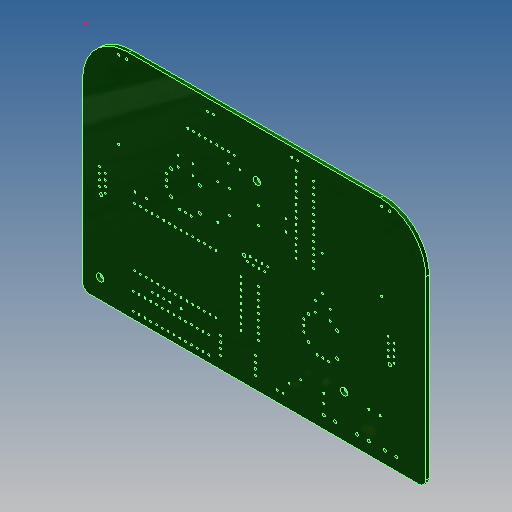
# Autodesk Inventor part: manette_2019.kicad_pcb_Contour
Saved by Autodesk Inventor 2019 (Build 230136000, 136)
## iProperties
Created: 2019-05-14
Part Number: manette_2019.kicad_pcb_Contour
Project: Nom Projet
Material: .
Description: Nom pièce
Document SubType Name: Modeling
Designer: Adel.KAHRIMANOVIC
Authority: brut Ø
Density: 0.001 g/cm^3
Appearance: Contour du circuit imprimé
Author: Adel.KAHRIMANOVIC
Material number: ---
Autodesk Inventor part; units mm, degrees
ref_plane "Plan YZ" through (0, 0, 0) normal (1, 0, 0) x (0, 1, 0)
ref_plane "Plan XZ" through (0, 0, 0) normal (0, 1, 0) x (-1, 0, 0)
ref_plane "Plan XY" through (0, 0, 0) normal (0, 0, 1) x (1, 0, 0)
sketch "Esquisse1" plane through (0, 0, 0) normal (0, 0, 1) x (1, 0, 0)
  point P0 (0, 0)
sketch "Esquisse6" plane through (0, 0, 0) normal (0, 0, 1) x (1, 0, 0)
  arc A0 (0, -97) -> (3, -100) centre (3, -97) ccw
  line L0 (3, -100) -> (147, -100)
  arc A1 (147, -100) -> (150, -97) centre (147, -97) ccw
  line L1 (150, -97) -> (150, -20)
  arc A2 (150, -20) -> (130, 0) centre (130, -20) ccw
  line L2 (130, 0) -> (20, 0)
  arc A3 (20, 0) -> (0, -20) centre (20, -20) ccw
  line L3 (0, -20) -> (0, -97)
  circle A4 centre (125.095, -82.55) radius 0.4
  circle A5 centre (130.095, -82.55) radius 0.4
  circle A6 centre (27.86, -51.435) radius 0.4
  circle A7 centre (22.86, -51.435) radius 0.4
  circle A8 centre (88.9, -28.575) radius 0.4
  circle A9 centre (88.9, -33.575) radius 0.4
  circle A10 centre (38.1165, -85.5345) radius 0.4
  circle A11 centre (43.1165, -85.5345) radius 0.4
  circle A12 centre (63.7667, -20.0406) radius 0.4
  circle A13 centre (68.7667, -20.0406) radius 0.4
  circle A14 centre (64.135, -29.5494) radius 0.4
  circle A15 centre (64.135, -39.7094) radius 0.4
  circle A16 centre (95.25, -86.36) radius 0.4
  circle A17 centre (105.41, -86.36) radius 0.4
  circle A18 centre (120.015, -94.615) radius 0.65
  circle A19 centre (125.095, -94.615) radius 0.65
  circle A20 centre (132.08, -94.615) radius 0.65
  circle A21 centre (137.16, -94.615) radius 0.65
  circle A22 centre (57.15, -5) radius 0.4
  circle A23 centre (54.61, -5) radius 0.4
  circle A24 centre (91.46, -4) radius 0.4
  circle A25 centre (94, -4) radius 0.4
  circle A26 centre (66.294, -15.748) radius 0.4
  circle A27 centre (63.754, -15.748) radius 0.4
  circle A28 centre (61.214, -15.748) radius 0.4
  circle A29 centre (58.674, -15.748) radius 0.4
  circle A30 centre (56.134, -15.748) radius 0.4
  circle A31 centre (53.594, -15.748) radius 0.4
  circle A32 centre (51.054, -15.748) radius 0.4
  circle A33 centre (48.514, -15.748) radius 0.4
  circle A34 centre (45.974, -15.748) radius 0.4
  circle A35 centre (105.41, -94.615) radius 0.65
  circle A36 centre (110.49, -94.615) radius 0.65
  circle A37 centre (87.63, -95.25) radius 0.4
  circle A38 centre (85.09, -95.25) radius 0.4
  circle A39 centre (136.144, -59.69) radius 0.4
  circle A40 centre (133.604, -58.42) radius 0.4
  circle A41 centre (136.144, -57.15) radius 0.4
  circle A42 centre (133.604, -55.88) radius 0.4
  circle A43 centre (136.144, -54.61) radius 0.4
  circle A44 centre (133.604, -53.34) radius 0.4
  circle A45 centre (136.144, -52.07) radius 0.4
  circle A46 centre (133.604, -50.8) radius 0.4
  circle A47 centre (9.906, -58.42) radius 0.4
  circle A48 centre (7.366, -57.15) radius 0.4
  circle A49 centre (9.906, -55.88) radius 0.4
  circle A50 centre (7.366, -54.61) radius 0.4
  circle A51 centre (9.906, -53.34) radius 0.4
  circle A52 centre (7.366, -52.07) radius 0.4
  circle A53 centre (9.906, -50.8) radius 0.4
  circle A54 centre (7.366, -49.53) radius 0.4
  circle A55 centre (80.9244, -50.73) radius 0.4
  circle A56 centre (79.6544, -53.27) radius 0.4
  circle A57 centre (78.3844, -50.73) radius 0.4
  circle A58 centre (77.1144, -53.27) radius 0.4
  circle A59 centre (75.8444, -50.73) radius 0.4
  circle A60 centre (74.5744, -53.27) radius 0.4
  circle A61 centre (73.3044, -50.73) radius 0.4
  circle A62 centre (72.0344, -53.27) radius 0.4
  circle A63 centre (36.75, -37.5) radius 0.45
  circle A64 centre (36.75, -40) radius 0.45
  circle A65 centre (36.75, -42.5) radius 0.45
  circle A66 centre (45, -48.25) radius 0.45
  circle A67 centre (42.5, -48.25) radius 0.45
  circle A68 centre (47.5, -48.25) radius 0.45
  circle A69 centre (41.75, -32.55) radius 0.4
  circle A70 centre (48.25, -32.55) radius 0.4
  circle A71 centre (48.25, -28.05) radius 0.4
  circle A72 centre (41.75, -28.05) radius 0.4
  circle A73 centre (101.75, -53.05) radius 0.4
  circle A74 centre (108.25, -53.05) radius 0.4
  circle A75 centre (108.25, -57.55) radius 0.4
  circle A76 centre (101.75, -57.55) radius 0.4
  circle A77 centre (107.5, -73.25) radius 0.45
  circle A78 centre (102.5, -73.25) radius 0.45
  circle A79 centre (105, -73.25) radius 0.45
  circle A80 centre (96.75, -67.5) radius 0.45
  circle A81 centre (96.75, -65) radius 0.45
  circle A82 centre (96.75, -62.5) radius 0.45
  circle A83 centre (76.835, -29.5494) radius 0.4
  circle A84 centre (76.835, -37.1694) radius 0.4
  circle A85 centre (90.17, -90.17) radius 0.4
  circle A86 centre (105.41, -90.17) radius 0.4
  circle A87 centre (59.055, -44.7894) radius 0.4
  circle A88 centre (59.055, -29.5494) radius 0.4
  circle A89 centre (104.775, -33.655) radius 0.4
  circle A90 centre (104.775, -48.895) radius 0.4
  circle A91 centre (15.75, -3) radius 0.5
  circle A92 centre (19.25, -3) radius 0.5
  circle A93 centre (15.75, -37) radius 0.5
  circle A94 centre (130.75, -3) radius 0.5
  circle A95 centre (134.25, -3) radius 0.5
  circle A96 centre (130.75, -37) radius 0.5
  circle A97 centre (37.975, -81.33) radius 0.4
  circle A98 centre (22.735, -81.33) radius 0.4
  circle A99 centre (53.215, -81.33) radius 0.4
  circle A100 centre (25.275, -81.33) radius 0.4
  circle A101 centre (40.515, -81.33) radius 0.4
  circle A102 centre (48.135, -81.33) radius 0.4
  circle A103 centre (27.815, -81.33) radius 0.4
  circle A104 centre (32.895, -81.33) radius 0.4
  circle A105 centre (43.055, -81.33) radius 0.4
  circle A106 centre (50.675, -81.33) radius 0.4
  circle A107 centre (55.755, -81.33) radius 0.4
  circle A108 centre (35.435, -81.33) radius 0.4
  circle A109 centre (45.595, -81.33) radius 0.4
  circle A110 centre (30.355, -81.33) radius 0.4
  circle A111 centre (58.295, -81.33) radius 0.4
  circle A112 centre (22.735, -55.83) radius 0.4
  circle A113 centre (25.275, -55.83) radius 0.4
  circle A114 centre (27.815, -55.83) radius 0.4
  circle A115 centre (30.355, -55.83) radius 0.4
  circle A116 centre (32.895, -55.83) radius 0.4
  circle A117 centre (35.435, -55.83) radius 0.4
  circle A118 centre (37.975, -55.83) radius 0.4
  circle A119 centre (40.515, -55.83) radius 0.4
  circle A120 centre (43.055, -55.83) radius 0.4
  circle A121 centre (45.595, -55.83) radius 0.4
  circle A122 centre (48.135, -55.83) radius 0.4
  circle A123 centre (50.675, -55.83) radius 0.4
  circle A124 centre (53.215, -55.83) radius 0.4
  circle A125 centre (55.755, -55.83) radius 0.4
  circle A126 centre (58.295, -55.83) radius 0.4
  circle A127 centre (55.1815, -96.9645) radius 0.4
  circle A128 centre (22.1615, -89.3445) radius 0.4
  circle A129 centre (52.6415, -96.9645) radius 0.4
  circle A130 centre (24.7015, -89.3445) radius 0.4
  circle A131 centre (50.1015, -96.9645) radius 0.4
  circle A132 centre (27.2415, -89.3445) radius 0.4
  circle A133 centre (47.5615, -96.9645) radius 0.4
  circle A134 centre (29.7815, -89.3445) radius 0.4
  circle A135 centre (45.0215, -96.9645) radius 0.4
  circle A136 centre (32.3215, -89.3445) radius 0.4
  circle A137 centre (42.4815, -96.9645) radius 0.4
  circle A138 centre (34.8615, -89.3445) radius 0.4
  circle A139 centre (39.9415, -96.9645) radius 0.4
  circle A140 centre (37.4015, -89.3445) radius 0.4
  circle A141 centre (37.4015, -96.9645) radius 0.4
  circle A142 centre (39.9415, -89.3445) radius 0.4
  circle A143 centre (34.8615, -96.9645) radius 0.4
  circle A144 centre (42.4815, -89.3445) radius 0.4
  circle A145 centre (32.3215, -96.9645) radius 0.4
  circle A146 centre (45.0215, -89.3445) radius 0.4
  circle A147 centre (29.7815, -96.9645) radius 0.4
  circle A148 centre (47.5615, -89.3445) radius 0.4
  circle A149 centre (27.2415, -96.9645) radius 0.4
  circle A150 centre (50.1015, -89.3445) radius 0.4
  circle A151 centre (24.7015, -96.9645) radius 0.4
  circle A152 centre (52.6415, -89.3445) radius 0.4
  circle A153 centre (22.1615, -96.9645) radius 0.4
  circle A154 centre (55.1815, -89.3445) radius 0.4
  circle A155 centre (93.345, -8.255) radius 0.4
  circle A156 centre (100.965, -41.275) radius 0.4
  circle A157 centre (93.345, -10.795) radius 0.4
  circle A158 centre (100.965, -38.735) radius 0.4
  circle A159 centre (93.345, -13.335) radius 0.4
  circle A160 centre (100.965, -36.195) radius 0.4
  circle A161 centre (93.345, -15.875) radius 0.4
  circle A162 centre (100.965, -33.655) radius 0.4
  circle A163 centre (93.345, -18.415) radius 0.4
  circle A164 centre (100.965, -31.115) radius 0.4
  circle A165 centre (93.345, -20.955) radius 0.4
  circle A166 centre (100.965, -28.575) radius 0.4
  circle A167 centre (93.345, -23.495) radius 0.4
  circle A168 centre (100.965, -26.035) radius 0.4
  circle A169 centre (93.345, -26.035) radius 0.4
  circle A170 centre (100.965, -23.495) radius 0.4
  circle A171 centre (93.345, -28.575) radius 0.4
  circle A172 centre (100.965, -20.955) radius 0.4
  circle A173 centre (93.345, -31.115) radius 0.4
  circle A174 centre (100.965, -18.415) radius 0.4
  circle A175 centre (93.345, -33.655) radius 0.4
  circle A176 centre (100.965, -15.875) radius 0.4
  circle A177 centre (93.345, -36.195) radius 0.4
  circle A178 centre (100.965, -13.335) radius 0.4
  circle A179 centre (93.345, -38.735) radius 0.4
  circle A180 centre (100.965, -10.795) radius 0.4
  circle A181 centre (93.345, -41.275) radius 0.4
  circle A182 centre (100.965, -8.255) radius 0.4
  circle A183 centre (69.215, -60.325) radius 0.4
  circle A184 centre (76.835, -80.645) radius 0.4
  circle A185 centre (69.215, -62.865) radius 0.4
  circle A186 centre (76.835, -78.105) radius 0.4
  circle A187 centre (69.215, -65.405) radius 0.4
  circle A188 centre (76.835, -75.565) radius 0.4
  circle A189 centre (69.215, -67.945) radius 0.4
  circle A190 centre (76.835, -73.025) radius 0.4
  circle A191 centre (69.215, -70.485) radius 0.4
  circle A192 centre (76.835, -70.485) radius 0.4
  circle A193 centre (69.215, -73.025) radius 0.4
  circle A194 centre (76.835, -67.945) radius 0.4
  circle A195 centre (69.215, -75.565) radius 0.4
  circle A196 centre (76.835, -65.405) radius 0.4
  circle A197 centre (69.215, -78.105) radius 0.4
  circle A198 centre (76.835, -62.865) radius 0.4
  circle A199 centre (69.215, -80.645) radius 0.4
  circle A200 centre (76.835, -60.325) radius 0.4
  circle A201 centre (60.325, -86.995) radius 0.45
  circle A202 centre (60.325, -89.535) radius 0.45
  circle A203 centre (60.325, -92.075) radius 0.45
  circle A204 centre (60.325, -94.615) radius 0.45
  circle A205 centre (75.565, -94.615) radius 0.45
  circle A206 centre (75.565, -92.075) radius 0.45
  circle A207 centre (75.565, -89.535) radius 0.45
  circle A208 centre (75.565, -86.995) radius 0.45
  circle A209 centre (30.4165, -85.5345) radius 0.4
  circle A210 centre (32.9165, -85.5345) radius 0.4
  circle A211 centre (35.4165, -85.5345) radius 0.4
  circle A212 centre (134.344, -61.09) radius 0.75
  circle A213 centre (8.106, -59.82) radius 0.75
  circle A214 centre (70.6344, -51.47) radius 0.75
  circle A215 centre (38.75, -34.7) radius 0.65
  circle A216 centre (38.75, -45.3) radius 0.65
  circle A217 centre (51.25, -45.3) radius 0.65
  circle A218 centre (51.25, -34.7) radius 0.65
  circle A219 centre (111.25, -59.7) radius 0.65
  circle A220 centre (111.25, -70.3) radius 0.65
  circle A221 centre (98.75, -70.3) radius 0.65
  circle A222 centre (98.75, -59.7) radius 0.65
  circle A223 centre (7.62, -91.44) radius 1.6
  circle A224 centre (114.3, -81.28) radius 1.6
  circle A225 centre (76.2, -20.5867) radius 1.6
  constraints: 226 centre point, 8 end point, 8 point on circle
extrude "manette_2019.kicad_pcb_Contour" add sketch "Esquisse6" along normal blind 1.6
